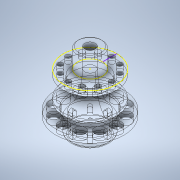
# Autodesk Inventor part: nsf_franke_bvr_diff
Saved by Autodesk Inventor 2020 (Build 240168000, 168)
## iProperties
Created: 2023-10-27
Part Number: nsf_franke_bvr_diff
Material: Типовые
Document SubType Name: Modeling
Designer: Сёма Пекуров
Density: 1 g/cm^3
Appearance: По умолчанию
Author: Сёма Пекуров
Autodesk Inventor part; units mm, degrees
ref_plane "XZ Plane" through (0, 0, 0) normal (0, 1, 0) x (-1, 0, 0)
ref_plane "XY Plane" through (0, 0, 0) normal (0, 0, 1) x (1, 0, 0)
sketch "Эскиз1" plane through (0, 0, 0) normal (0, 1, 0) x (-1, 0, 0)
  circle A0 centre (0, 0) radius 7.35
  dimension "d0" = 14.7
  constraints: 1 centre point, 1 coincident
  measures "d0" diameter of A0
extrude "Выдавливание1" add sketch "Эскиз1" along normal blind 2
sketch "Эскиз2" plane through (0, 2, 0) normal (0, 1, 0) x (1, 0, 0)
  circle A0 centre (0, 0) radius 7.35
  circle A1 centre (0, 0) radius 6
  dimension "d3" = 12
  constraints: 2 centre point, 2 coincident
  measures "d3" diameter of A1
extrude "Выдавливание2" add sketch "Эскиз2" along normal blind 4
ref_plane "РабПлоскость1" through (7.35, 0, 0) normal (1, 0, 0) x (0, 1, 0)
sketch "Эскиз3" plane through (7.35, 0, 0) normal (1, 0, 0) x (0, 1, 0)
  line L0 (2, -6) -> (2, 6) projected
  line L1 (2, 0) -> (0, 0)
  line L2 (4, 0) -> (2, 0) construction
  line L3 (4, 0.8) -> (1.75, 0.8)
  line L4 (1.75, -0.8) -> (4, -0.8)
  arc A0 (4, -0.8) -> (4, 0.8) centre (4, 0) ccw
  line L5 (1.75, 0.8) -> (1.75, -0.8)
  point P0 (3, 0)
  point P1 (2, 0.8)
  point P2 (2, -0.8)
  dimension "d7" = 2
  dimension "d8" = 0.8
  constraints: 12 end point, 2 midpoint, 2 parallel, 2 point on circle, 2 tangent, 1 centre point, 1 collinear, 1 horizontal
  measures "d7" distance of L1.start L2.start
  measures "d8" distance from line of L4 point (3, 0)
extrude "Выдавливание3" cut sketch "Эскиз3" against normal up to surface contours L0 L3 A0 L4 round surface about axis through (0, 2, 0) along (0, 1, 0) radius 6 far side no
pattern_circular "Круговой массив1" count 8 over 360 about axis through (0, -10, 0) along (0, 1, 0) of "Выдавливание3"
sketch "Эскиз4" plane through (0, 6, 0) normal (0, 1, 0) x (1, 0, 0)
  circle A0 centre (0, 0) radius 12.95
  circle A1 centre (0, 0) radius 7.35 projected
  circle A2 centre (0, 0) radius 6
  dimension "d17" = 25.9
  constraints: 2 centre point, 2 coincident
  measures "d17" diameter of A0
extrude "Выдавливание4" add sketch "Эскиз4" along normal blind 2 contours A0 | A1
sketch "Эскиз5" plane through (0, 6, 0) normal (0, -1, 0) x (1, 0, 0)
  circle A0 centre (0, 0) radius 12.95 projected
  line L0 (0, -12.95) -> (0, -7.35)
  arc A1 (-0.8, -7.3063) -> (0.8, -7.3063) centre (0, 0) ccw projected
  circle A2 centre (0, -10.15) radius 2
  dimension "d20" = 4
  constraints: 2 end point, 1 centre point, 1 midpoint, 1 point on circle, 1 vertical, 1 vertical alignment, 1 other
  measures "d20" diameter of A2
extrude "Выдавливание5" cut sketch "Эскиз5" against normal up to next contours A2 L0 | L0 A2
pattern_circular "Круговой массив2" count 12 over 360 about axis through (0, -10, 0) along (0, 1, 0) of "Выдавливание5"
sketch "Эскиз6" plane through (0, 0, 0) normal (0, 0, 1) x (1, 0, 0)
  line L0 (8.15, 8) -> (12.15, 8) projected
  line L1 (8.15, 8) -> (0, 8)
  line L2 (7.35, 6) -> (-7.35, 6) projected
  line L3 (0, 6) -> (0, 21.5)
  line L4 (0, 21.5) -> (0, 19.5)
  line L5 (0, 19.5) -> (0, 17.5)
  line L6 (0, 8) -> (0, 9)
  line L7 (0, 9) -> (0, 11)
  line L8 (0, 11) -> (0, 12)
  line L9 (0, 12) -> (0, 17.5)
  line L10 (0, 17.5) -> (0, 12)
  line L11 (8.15, 8) -> (8.15, 9)
  line L12 (8.15, 9) -> (0, 9)
  line L13 (12.15, 8) -> (8.15, 8)
  line L14 (12.95, 6) -> (-12.95, 6) projected
  line L15 (0, 11) -> (10.15, 11)
  line L16 (10.15, 11) -> (8.15, 9)
  line L17 (10.15, 11) -> (10.15, 12)
  line L18 (10.15, 12) -> (0, 12)
  line L19 (0, 17.5) -> (6.5, 17.5)
  line L20 (12.95, 8) -> (-12.95, 8) projected
  line L21 (6.5, 17.5) -> (10.15, 12)
  line L22 (6.5, 17.5) -> (6.5, 19.5)
  line L23 (6.5, 19.5) -> (0, 19.5)
  line L24 (0, 21.5) -> (10.15, 21.5)
  line L25 (10.15, 21.5) -> (10.15, 19.5)
  line L26 (10.15, 19.5) -> (6.5, 19.5)
  line L27 (0, 21.5) -> (0, 29)
  line L28 (0, 29) -> (4.75, 29)
  line L29 (4.75, 29) -> (4.75, 21.5)
  line L30 (0, 29) -> (2, 29)
  line L31 (2, 29) -> (2, 21.5)
  line L32 (-6, 8) -> (6, 8) projected
  spline S0 degree 2 poles (2, 21.5) (2.5846, 4.5577) (12.95, 6) knots 0 0 0 1 1 1
  line L33 (0, -5.8) -> (0, 34.8) projected
  point P0 (0, 0)
  dimension "d26" = 15.5
  dimension "d27" = 2
  dimension "d28" = 2
  dimension "d29" = 1
  dimension "d30" = 2
  dimension "d31" = 1
  dimension "d32" = 5.5
  dimension "d33" = 6.5
  dimension "d34" = 7.5
  dimension "d35" = 4.75
  dimension "d36" = 2
  constraints: 56 end point, 9 point on line, 8 perpendicular, 4 horizontal, 4 vertical, 2 collinear, 2 parallel, 1 midpoint, 3 other
  measures "d26" distance of L3.start L3.end
  measures "d27" distance of L3.end L4.end
  measures "d28" distance of L4.end L5.end
  measures "d29" distance of L1.end L6.end
  measures "d30" distance of L6.end L7.end
  measures "d31" distance of L7.end L8.end
  measures "d32" distance of L8.end L5.end
  measures "d33" distance of L5.end L19.end
  measures "d34" distance of L3.end L27.end
  measures "d35" distance of L27.end L28.end
  measures "d36" distance of L27.end L30.end
revolve "Вращение1" add sketch "Эскиз6" angle 360 about axis through (0, -10, 0) along (0, 1, 0) contours L1 S0 L12 L11 | L12 S0 L15 L16 | L15 S0 L18 L17 | L18 S0 L19 L21 | L19 S0 L23 L22 | L23 S0 L24 L25 L26 | L31 L28 L29 L24
sketch "Эскиз7" plane through (0, 21.5, 0) normal (0, 1, 0) x (1, 0, 0)
  circle A0 centre (0, 0) radius 10.15 projected
  line L0 (0, 10.15) -> (0, 4.75)
  circle A1 centre (0, 0) radius 4.75 projected
  constraints: 2 end point, 2 vertical alignment, 1 vertical, 2 other
sketch "Эскиз8" plane through (0, 19.5, 0) normal (0, -1, 0) x (1, 0, 0)
  circle A0 centre (0, 0) radius 6.5 projected
  line L0 (0, -6.5) -> (0, -10.15)
  circle A1 centre (0, 0) radius 10.15 projected
  circle A2 centre (0, -8.325) radius 1
  dimension "d38" = 2
  constraints: 2 end point, 2 vertical alignment, 1 centre point, 1 midpoint, 1 vertical, 2 other
  measures "d38" diameter of A2
extrude "Выдавливание6" cut sketch "Эскиз8" against normal up to surface (2 mm away) contours A2 L0 | L0 A2
pattern_circular "Круговой массив3" count 12 over 360 about axis through (0, -10, 0) along (0, 1, 0) of "Выдавливание6"
sketch "Эскиз9" plane through (0, 0, 0) normal (1, 0, 0) x (0, 1, 0)
  line L0 (6, -7.35) -> (6, 7.35)
  line L1 (2, -7.3063) -> (2, -5.9464)
  line L2 (2, -7.3063) -> (2, 0)
  line L3 (2, 0) -> (6, 0)
  line L4 (12, 10.15) -> (12, -10.15)
  spline S0 degree 2 poles (2, -7.3063) (3.3807, -1.6096) (5.0539, -0.3545) knots 0 0 0 1 1 1
  line L5 (-5.8, 0) -> (34.8, 0)
  line L6 (2, 0) -> (4.8001, 0)
  arc A0 (5.0539, -0.3545) -> (5.236, 0) centre (4.8001, 0) ccw
  line L7 (3.9448, -1.1864) -> (6.1629, 0.4774) construction
  arc A1 (5.991, 0.0672) -> (4.3867, -1.1362) centre (6.462, -2.2317) ccw construction
  point P0 (0, 0)
  point P1 (5.236, 0)
  constraints: 8 end point, 3 midpoint, 3 point on circle, 2 centre point, 2 point on line, 1 coincident, 1 collinear, 1 perpendicular, 5 other
revolve "Вращение2" add sketch "Эскиз9" angle 360 about axis through (0, -10, 0) along (0, 1, 0)
chamfer "Фаска2" distance 0.5 angle 45 1 edges at (-4.75, 29, 0)
fillet "Сопряжение1" radius 1 1 edges at (7.35, 0, 0)
